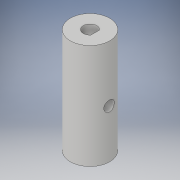
# Autodesk Inventor part: Motor_Spiral
Saved by Autodesk Inventor 2019 (Build 230136000, 136)
## iProperties
Created: 2021-06-02
Part Number: Motor_Spiral
Material: Generisch
Document SubType Name: Modeling
Designer: Bergi
Density: 1 g/cm^3
Appearance: Vorgabe
Author: Bergi
Autodesk Inventor part; units mm, degrees
ref_plane "YZ Plane" through (0, 0, 0) normal (1, 0, 0) x (0, 1, 0)
ref_plane "XZ Plane" through (0, 0, 0) normal (0, 1, 0) x (-1, 0, 0)
ref_plane "XY Plane" through (0, 0, 0) normal (0, 0, 1) x (1, 0, 0)
sketch "Skizze1" plane through (0, 0, 0) normal (0, 1, 0) x (-1, 0, 0)
  circle A0 centre (0, 0) radius 7.5
  dimension "d0" = 15
  constraints: 1 centre point, 1 coincident
  measures "d0" diameter of A0
extrude "Extrusion1" add sketch "Skizze1" along normal blind 40
sketch "Skizze2" plane through (0, 40, 0) normal (0, 1, 0) x (1, 0, 0)
  arc A0 (2, 1.6613) -> (2, -1.6613) centre (0, 0) ccw
  line L0 (2, -1.6613) -> (2, 1.6613)
  dimension "d3" = 5.2
  dimension "d4" = 4.6
  constraints: 2 end point, 2 point on circle, 1 centre point, 1 coincident, 1 vertical
  measures "d3" diameter of A0
extrude "Extrusion2" cut sketch "Skizze2" against normal blind 15
sketch "Skizze3" plane through (0, 0, 0) normal (1, 0, 0) x (0, 1, 0)
  line L0 (-8, 0) -> (48, 0) construction
  line L1 (40, -7.5) -> (40, 7.5) projected
  line L2 (0, 7.5) -> (0, -7.5) projected
  point P0 (0, 0)
  point P1 (18.5, 0)
  dimension "d7" = 21.5
  constraints: 1 point on line
  measures "d7" distance from line of L1 point (18.5, 0)
hole "Bohrung1" at (0, 18.5, 0) direction (-1, 0, 0) diameter 4 end through all both
